Autodesk Inventor part; units mm, degrees
(part 2 of 3)
sketch "Sketch14" plane through (0, 0, 0) normal (0, 1, 0) x (1, 0, 0)
  line L0 (-0.8228, 6.9318) -> (-0.8228, 38.6692) construction
  line L1 (-0.8228, 38.6692) -> (1.7801, 38.6692) construction
  line L2 (1.7801, 38.6692) -> (1.7801, 6.9318) construction
  line L3 (1.7801, 6.9318) -> (-0.8228, 6.9318) construction
  line L4 (-3.7716, 9.8924) -> (-3.7716, 35.0917) construction
  line L5 (-3.7716, 35.0917) -> (-1.431, 35.0917) construction
  line L6 (-1.431, 35.0917) -> (-1.431, 9.8924) construction
  line L7 (-1.431, 9.8924) -> (-3.7716, 9.8924) construction
  spline S0 degree 2 poles (-1.6938, 10.6525) (-1.6938, 10.4354) (-1.7845, 10.1307) (-1.8494, 9.9961) knots 0 0 0 1 2 2 2
  line L8 (-1.8494, 9.9961) -> (-2.1832, 9.9961)
  line L9 (-2.1832, 9.9961) -> (-2.1832, 10.0156)
  spline S1 degree 2 poles (-2.1832, 10.0156) (-2.06, 10.1469) (-1.9239, 10.4791) (-1.9239, 10.6331) knots 0 0 0 1 2 2 2
  spline S2 degree 2 poles (-1.9239, 10.6331) (-1.9239, 10.8535) (-2.1071, 11.0788) (-2.2578, 11.0788) knots 0 0 0 1 2 2 2
  spline S3 degree 2 poles (-2.2578, 11.0788) (-2.3777, 11.0788) (-2.5268, 10.9605) (-2.5641, 10.8324) knots 0 0 0 1 2 2 2
  spline S4 degree 2 poles (-2.5641, 10.8324) (-2.59, 10.7401) (-2.6257, 10.5861) (-2.6549, 10.471) knots 0 0 0 1 2 2 2
  spline S5 degree 2 poles (-2.6549, 10.471) (-2.6824, 10.3673) (-2.7651, 10.2036) (-2.8315, 10.1404) knots 0 0 0 1 2 2 2
  spline S6 degree 2 poles (-2.8315, 10.1404) (-2.898, 10.0788) (-3.0763, 10.0107) (-3.193, 10.0107) knots 0 0 0 1 2 2 2
  spline S7 degree 2 poles (-3.193, 10.0107) (-3.4361, 10.0107) (-3.7651, 10.39) (-3.7651, 10.6833) knots 0 0 0 1 2 2 2
  spline S8 degree 2 poles (-3.7651, 10.6833) (-3.7651, 10.8519) (-3.6986, 11.1501) (-3.6354, 11.2781) knots 0 0 0 1 2 2 2
  line L10 (-3.6354, 11.2781) -> (-3.3177, 11.2781)
  line L11 (-3.3177, 11.2781) -> (-3.3177, 11.2587)
  spline S9 degree 2 poles (-3.3177, 11.2587) (-3.4053, 11.1631) (-3.5349, 10.8649) (-3.5349, 10.7012) knots 0 0 0 1 2 2 2
  spline S10 degree 2 poles (-3.5349, 10.7012) (-3.5349, 10.5164) (-3.3615, 10.2879) (-3.2205, 10.2879) knots 0 0 0 1 2 2 2
  spline S11 degree 2 poles (-3.2205, 10.2879) (-3.0941, 10.2879) (-2.9434, 10.4224) (-2.9093, 10.5488) knots 0 0 0 1 2 2 2
  spline S12 degree 2 poles (-2.9093, 10.5488) (-2.8866, 10.6331) (-2.8283, 10.8778) (-2.804, 10.9589) knots 0 0 0 1 2 2 2
  spline S13 degree 2 poles (-2.804, 10.9589) (-2.7408, 11.1647) (-2.4863, 11.3559) (-2.2999, 11.3559) knots 0 0 0 1 2 2 2
  spline S14 degree 2 poles (-2.2999, 11.3559) (-2.1816, 11.3559) (-1.9547, 11.2603) (-1.8753, 11.1744) knots 0 0 0 1 2 2 2
  spline S15 degree 2 poles (-1.8753, 11.1744) (-1.7878, 11.0788) (-1.6938, 10.8357) (-1.6938, 10.6525) knots 0 0 0 1 2 2 2
  line L12 (-1.7294, 12.3235) -> (-1.7294, 11.5488)
  line L13 (-1.7294, 11.5488) -> (-1.9336, 11.5488)
  line L14 (-1.9336, 11.5488) -> (-1.9336, 11.8033)
  line L15 (-1.9336, 11.8033) -> (-3.5252, 11.8033)
  line L16 (-3.5252, 11.8033) -> (-3.5252, 11.5488)
  line L17 (-3.5252, 11.5488) -> (-3.7294, 11.5488)
  line L18 (-3.7294, 11.5488) -> (-3.7294, 12.3235)
  line L19 (-3.7294, 12.3235) -> (-3.5252, 12.3235)
  line L20 (-3.5252, 12.3235) -> (-3.5252, 12.0691)
  line L21 (-3.5252, 12.0691) -> (-1.9336, 12.0691)
  line L22 (-1.9336, 12.0691) -> (-1.9336, 12.3235)
  line L23 (-1.9336, 12.3235) -> (-1.7294, 12.3235)
  line L24 (-3.7294, 14.894) -> (-1.7294, 14.3916)
  line L25 (-1.7294, 14.3916) -> (-1.7294, 14.0934)
  line L26 (-1.7294, 14.0934) -> (-3.3891, 13.6866)
  line L27 (-3.3891, 13.6866) -> (-1.7294, 13.2911)
  line L28 (-1.7294, 13.2911) -> (-1.7294, 12.9961)
  line L29 (-1.7294, 12.9961) -> (-3.7294, 12.4856)
  line L30 (-3.7294, 12.4856) -> (-3.7294, 12.7595)
  line L31 (-3.7294, 12.7595) -> (-2.0714, 13.1615)
  line L32 (-2.0714, 13.1615) -> (-3.7294, 13.5602)
  line L33 (-3.7294, 13.5602) -> (-3.7294, 13.8308)
  line L34 (-3.7294, 13.8308) -> (-2.0519, 14.2328)
  line L35 (-2.0519, 14.2328) -> (-3.7294, 14.6331)
  line L36 (-3.7294, 14.6331) -> (-3.7294, 14.894)
  line L37 (-1.7294, 14.9167) -> (-3.7294, 15.5909)
  line L38 (-3.7294, 15.5909) -> (-3.7294, 15.9183)
  line L39 (-3.7294, 15.9183) -> (-1.7294, 16.5926)
  line L40 (-1.7294, 16.5926) -> (-1.7294, 16.3122)
  line L41 (-1.7294, 16.3122) -> (-2.2886, 16.1307)
  line L42 (-2.2886, 16.1307) -> (-2.2886, 15.3673)
  line L43 (-2.2886, 15.3673) -> (-1.7294, 15.1858)
  line L44 (-1.7294, 15.1858) -> (-1.7294, 14.9167)
  line L45 (-2.5155, 16.0577) -> (-3.4571, 15.7482)
  line L46 (-3.4571, 15.7482) -> (-2.5155, 15.4402)
  line L47 (-2.5155, 15.4402) -> (-2.5155, 16.0577)
  line L48 (-1.7294, 17.249) -> (-3.4928, 17.249)
  line L49 (-3.4928, 17.249) -> (-3.4928, 16.578)
  line L50 (-3.4928, 16.578) -> (-3.7294, 16.578)
  line L51 (-3.7294, 16.578) -> (-3.7294, 18.1858)
  line L52 (-3.7294, 18.1858) -> (-3.4928, 18.1858)
  line L53 (-3.4928, 18.1858) -> (-3.4928, 17.5148)
  line L54 (-3.4928, 17.5148) -> (-1.7294, 17.5148)
  line L55 (-1.7294, 17.5148) -> (-1.7294, 17.249)
  line L56 (-1.7294, 19.9443) -> (-1.7294, 19.1696)
  line L57 (-1.7294, 19.1696) -> (-1.9336, 19.1696)
  line L58 (-1.9336, 19.1696) -> (-1.9336, 19.424)
  line L59 (-1.9336, 19.424) -> (-3.5252, 19.424)
  line L60 (-3.5252, 19.424) -> (-3.5252, 19.1696)
  line L61 (-3.5252, 19.1696) -> (-3.7294, 19.1696)
  line L62 (-3.7294, 19.1696) -> (-3.7294, 19.9443)
  line L63 (-3.7294, 19.9443) -> (-3.5252, 19.9443)
  line L64 (-3.5252, 19.9443) -> (-3.5252, 19.6898)
  line L65 (-3.5252, 19.6898) -> (-1.9336, 19.6898)
  line L66 (-1.9336, 19.6898) -> (-1.9336, 19.9443)
  line L67 (-1.9336, 19.9443) -> (-1.7294, 19.9443)
  line L68 (-1.7294, 21.7044) -> (-1.7294, 21.4062)
  line L69 (-1.7294, 21.4062) -> (-3.4539, 20.5213)
  line L70 (-3.4539, 20.5213) -> (-1.7294, 20.5213)
  line L71 (-1.7294, 20.5213) -> (-1.7294, 20.2733)
  line L72 (-1.7294, 20.2733) -> (-3.7294, 20.2733)
  line L73 (-3.7294, 20.2733) -> (-3.7294, 20.6509)
  line L74 (-3.7294, 20.6509) -> (-2.1459, 21.4564)
  line L75 (-2.1459, 21.4564) -> (-3.7294, 21.4564)
  line L76 (-3.7294, 21.4564) -> (-3.7294, 21.7044)
  line L77 (-3.7294, 21.7044) -> (-1.7294, 21.7044)
  spline S16 degree 2 poles (-1.6938, 22.8908) (-1.6938, 22.6963) (-1.825, 22.3673) (-1.9563, 22.2473) knots 0 0 0 1 2 2 2
  spline S17 degree 2 poles (-1.9563, 22.2473) (-2.086, 22.1274) (-2.475, 21.9961) (-2.7278, 21.9961) knots 0 0 0 1 2 2 2
  spline S18 degree 2 poles (-2.7278, 21.9961) (-2.979, 21.9961) (-3.3518, 22.1242) (-3.4895, 22.2457) knots 0 0 0 1 2 2 2
  spline S19 degree 2 poles (-3.4895, 22.2457) (-3.6241, 22.3657) (-3.7651, 22.6931) (-3.7651, 22.8956) knots 0 0 0 1 2 2 2
  spline S20 degree 2 poles (-3.7651, 22.8956) (-3.7651, 22.9961) (-3.7359, 23.1728) (-3.7132, 23.2473) knots 0 0 0 1 2 2 2
  spline S21 degree 2 poles (-3.7132, 23.2473) (-3.6921, 23.3122) (-3.6322, 23.4467) (-3.5965, 23.5132) knots 0 0 0 1 2 2 2
  line L78 (-3.5965, 23.5132) -> (-3.2756, 23.5132)
  line L79 (-3.2756, 23.5132) -> (-3.2756, 23.4921)
  spline S22 degree 2 poles (-3.2756, 23.4921) (-3.308, 23.4564) (-3.3988, 23.3462) (-3.4425, 23.2668) knots 0 0 0 1 2 2 2
  spline S23 degree 2 poles (-3.4425, 23.2668) (-3.4847, 23.1906) (-3.5382, 23.0107) (-3.5382, 22.894) knots 0 0 0 1 2 2 2
  spline S24 degree 2 poles (-3.5382, 22.894) (-3.5382, 22.766) (-3.4328, 22.5375) (-3.3323, 22.4516) knots 0 0 0 1 2 2 2
  spline S25 degree 2 poles (-3.3323, 22.4516) (-3.2302, 22.3673) (-2.9207, 22.2733) (-2.7278, 22.2733) knots 0 0 0 1 2 2 2
  spline S26 degree 2 poles (-2.7278, 22.2733) (-2.522, 22.2733) (-2.2254, 22.3721) (-2.1233, 22.458) knots 0 0 0 1 2 2 2
  spline S27 degree 2 poles (-2.1233, 22.458) (-2.0244, 22.5423) (-1.9239, 22.7676) (-1.9239, 22.894) knots 0 0 0 1 2 2 2
  spline S28 degree 2 poles (-1.9239, 22.894) (-1.9239, 23.0091) (-1.9806, 23.2052) (-2.0228, 23.2814) knots 0 0 0 1 2 2 2
  spline S29 degree 2 poles (-2.0228, 23.2814) (-2.0649, 23.3543) (-2.1524, 23.4629) (-2.1832, 23.4937) knots 0 0 0 1 2 2 2
  line L80 (-2.1832, 23.4937) -> (-2.1832, 23.5132)
  line L81 (-2.1832, 23.5132) -> (-1.8656, 23.5132)
  spline S30 degree 2 poles (-1.8656, 23.5132) (-1.8348, 23.4467) (-1.778, 23.33) (-1.7521, 23.2473) knots 0 0 0 1 2 2 2
  spline S31 degree 2 poles (-1.7521, 23.2473) (-1.7229, 23.1598) (-1.6938, 23.0107) (-1.6938, 22.8908) knots 0 0 0 1 2 2 2
  spline S32 degree 2 poles (-1.24, 26.2814) (-1.2221, 26.2085) (-1.2027, 26.0496) (-1.2027, 25.9702) knots 0 0 0 1 2 2 2
  spline S33 degree 2 poles (-1.2027, 25.9702) (-1.2027, 25.7449) (-1.4539, 25.4645) (-1.6873, 25.4516) knots 0 0 0 1 2 2 2
  spline S34 degree 2 poles (-1.6873, 25.4516) (-1.6873, 25.4337) (-1.6873, 25.4029) (-1.6873, 25.39) knots 0 0 0 1 2 2 2
  spline S35 degree 2 poles (-1.6873, 25.39) (-1.6873, 25.1874) (-1.825, 24.8616) (-1.9596, 24.7449) knots 0 0 0 1 2 2 2
  spline S36 degree 2 poles (-1.9596, 24.7449) (-2.0925, 24.6298) (-2.4814, 24.5067) (-2.7278, 24.5067) knots 0 0 0 1 2 2 2
  spline S37 degree 2 poles (-2.7278, 24.5067) (-2.9806, 24.5067) (-3.3631, 24.6315) (-3.4993, 24.7465) knots 0 0 0 1 2 2 2
  spline S38 degree 2 poles (-3.4993, 24.7465) (-3.6338, 24.8632) (-3.7716, 25.189) (-3.7716, 25.39) knots 0 0 0 1 2 2 2
  spline S39 degree 2 poles (-3.7716, 25.39) (-3.7716, 25.5942) (-3.6289, 25.9216) (-3.4993, 26.035) knots 0 0 0 1 2 2 2
  spline S40 degree 2 poles (-3.4993, 26.035) (-3.368, 26.1485) (-2.9774, 26.2749) (-2.7278, 26.2749) knots 0 0 0 1 2 2 2
  spline S41 degree 2 poles (-2.7278, 26.2749) (-2.3388, 26.2749) (-1.8331, 25.9718) (-1.744, 25.7076) knots 0 0 0 1 2 2 2
  spline S42 degree 2 poles (-1.744, 25.7076) (-1.6694, 25.7141) (-1.5495, 25.753) (-1.5155, 25.7838) knots 0 0 0 1 2 2 2
  spline S43 degree 2 poles (-1.5155, 25.7838) (-1.4733, 25.8211) (-1.4344, 25.9232) (-1.4344, 26.014) knots 0 0 0 1 2 2 2
  spline S44 degree 2 poles (-1.4344, 26.014) (-1.4344, 26.0674) (-1.4685, 26.2133) (-1.4814, 26.2457) knots 0 0 0 1 2 2 2
  line L82 (-1.4814, 26.2457) -> (-1.4814, 26.2814)
  line L83 (-1.4814, 26.2814) -> (-1.24, 26.2814)
  spline S45 degree 2 poles (-2.7278, 25.9978) (-2.9271, 25.9978) (-3.2335, 25.9119) (-3.334, 25.8341) knots 0 0 0 1 2 2 2
  spline S46 degree 2 poles (-3.334, 25.8341) (-3.4377, 25.7546) (-3.5414, 25.531) (-3.5414, 25.3916) knots 0 0 0 1 2 2 2
  spline S47 degree 2 poles (-3.5414, 25.3916) (-3.5414, 25.2473) (-3.4409, 25.0302) (-3.334, 24.9475) knots 0 0 0 1 2 2 2
  spline S48 degree 2 poles (-3.334, 24.9475) (-3.2318, 24.8681) (-2.9223, 24.7838) (-2.7278, 24.7838) knots 0 0 0 1 2 2 2
  spline S49 degree 2 poles (-2.7278, 24.7838) (-2.334, 24.7838) (-1.9142, 25.1144) (-1.9142, 25.3916) knots 0 0 0 1 2 2 2
  spline S50 degree 2 poles (-1.9142, 25.3916) (-1.9142, 25.6687) (-2.334, 25.9978) (-2.7278, 25.9978) knots 0 0 0 1 2 2 2
  spline S51 degree 2 poles (-3.5398, 27.0496) (-3.5398, 26.9767) (-3.5041, 26.8324) (-3.4766, 26.7627) knots 0 0 0 1 2 2 2
  spline S52 degree 2 poles (-3.4766, 26.7627) (-3.449, 26.6979) (-3.3907, 26.6023) (-3.3647, 26.565) knots 0 0 0 1 2 2 2
  line L84 (-3.3647, 26.565) -> (-3.3647, 26.5488)
  line L85 (-3.3647, 26.5488) -> (-3.6484, 26.5488)
  spline S53 degree 2 poles (-3.6484, 26.5488) (-3.6954, 26.6363) (-3.7716, 26.9362) (-3.7716, 27.0707) knots 0 0 0 1 2 2 2
  spline S54 degree 2 poles (-3.7716, 27.0707) (-3.7716, 27.2068) (-3.7165, 27.4094) (-3.6581, 27.4921) knots 0 0 0 1 2 2 2
  spline S55 degree 2 poles (-3.6581, 27.4921) (-3.5949, 27.5796) (-3.4118, 27.6704) (-3.2886, 27.6704) knots 0 0 0 1 2 2 2
  spline S56 degree 2 poles (-3.2886, 27.6704) (-3.1233, 27.6704) (-2.8737, 27.4532) (-2.8412, 27.3008) knots 0 0 0 1 2 2 2
  line L86 (-2.8412, 27.3008) -> (-2.8218, 27.3008)
  spline S57 degree 2 poles (-2.8218, 27.3008) (-2.8088, 27.364) (-2.7505, 27.5083) (-2.6921, 27.5699) knots 0 0 0 1 2 2 2
  spline S58 degree 2 poles (-2.6921, 27.5699) (-2.6354, 27.6315) (-2.4539, 27.7093) (-2.3226, 27.7093) knots 0 0 0 1 2 2 2
  spline S59 degree 2 poles (-2.3226, 27.7093) (-2.1881, 27.7093) (-1.9596, 27.6169) (-1.872, 27.5326) knots 0 0 0 1 2 2 2
  spline S60 degree 2 poles (-1.872, 27.5326) (-1.7813, 27.4451) (-1.6873, 27.1971) (-1.6873, 27.0399) knots 0 0 0 1 2 2 2
  spline S61 degree 2 poles (-1.6873, 27.0399) (-1.6873, 26.8892) (-1.7602, 26.5942) (-1.8105, 26.4937) knots 0 0 0 1 2 2 2
  line L87 (-1.8105, 26.4937) -> (-2.0941, 26.4937)
  line L88 (-2.0941, 26.4937) -> (-2.0941, 26.5132)
  spline S62 degree 2 poles (-2.0941, 26.5132) (-2.0325, 26.5974) (-1.919, 26.8827) (-1.919, 27.0237) knots 0 0 0 1 2 2 2
  spline S63 degree 2 poles (-1.919, 27.0237) (-1.919, 27.1063) (-1.9709, 27.2717) (-2.0309, 27.3268) knots 0 0 0 1 2 2 2
  spline S64 degree 2 poles (-2.0309, 27.3268) (-2.0908, 27.3803) (-2.2335, 27.437) (-2.3421, 27.437) knots 0 0 0 1 2 2 2
  spline S65 degree 2 poles (-2.3421, 27.437) (-2.4506, 27.437) (-2.5917, 27.3738) (-2.6322, 27.317) knots 0 0 0 1 2 2 2
  spline S66 degree 2 poles (-2.6322, 27.317) (-2.6727, 27.2603) (-2.7035, 27.1063) (-2.7035, 27.0156) knots 0 0 0 1 2 2 2
  line L89 (-2.7035, 27.0156) -> (-2.7035, 26.9021)
  line L90 (-2.7035, 26.9021) -> (-2.9255, 26.9021)
  line L91 (-2.9255, 26.9021) -> (-2.9255, 26.9913)
  spline S67 degree 2 poles (-2.9255, 26.9913) (-2.9255, 27.1712) (-3.0973, 27.3981) (-3.261, 27.3981) knots 0 0 0 1 2 2 2
  spline S68 degree 2 poles (-3.261, 27.3981) (-3.3372, 27.3981) (-3.4458, 27.3397) (-3.4782, 27.2927) knots 0 0 0 1 2 2 2
  spline S69 degree 2 poles (-3.4782, 27.2927) (-3.5122, 27.2425) (-3.5398, 27.1193) (-3.5398, 27.0496) knots 0 0 0 1 2 2 2
  line L92 (-1.7294, 30.1031) -> (-1.7294, 28.8697)
  line L93 (-1.7294, 28.8697) -> (-2.013, 28.8697)
  spline S70 degree 2 poles (-2.013, 28.8697) (-2.1378, 29.0026) (-2.3696, 29.2392) (-2.4944, 29.3527) knots 0 0 0 1 2 2 2
  spline S71 degree 2 poles (-2.4944, 29.3527) (-2.7456, 29.5812) (-3.0471, 29.7482) (-3.2075, 29.7482) knots 0 0 0 1 2 2 2
  spline S72 degree 2 poles (-3.2075, 29.7482) (-3.2918, 29.7482) (-3.4182, 29.6963) (-3.4588, 29.6493) knots 0 0 0 1 2 2 2
  spline S73 degree 2 poles (-3.4588, 29.6493) (-3.4993, 29.6023) (-3.5398, 29.4791) (-3.5398, 29.4046) knots 0 0 0 1 2 2 2
  spline S74 degree 2 poles (-3.5398, 29.4046) (-3.5398, 29.3332) (-3.5041, 29.1874) (-3.4766, 29.1209) knots 0 0 0 1 2 2 2
  spline S75 degree 2 poles (-3.4766, 29.1209) (-3.4539, 29.0642) (-3.3891, 28.9589) (-3.3664, 28.9264) knots 0 0 0 1 2 2 2
  line L94 (-3.3664, 28.9264) -> (-3.3664, 28.9119)
  line L95 (-3.3664, 28.9119) -> (-3.6516, 28.9119)
  spline S76 degree 2 poles (-3.6516, 28.9119) (-3.6921, 28.9945) (-3.7716, 29.2911) (-3.7716, 29.424) knots 0 0 0 1 2 2 2
  spline S77 degree 2 poles (-3.7716, 29.424) (-3.7716, 29.7044) (-3.475, 30.0204) (-3.2221, 30.0204) knots 0 0 0 1 2 2 2
  spline S78 degree 2 poles (-3.2221, 30.0204) (-3.1038, 30.0204) (-2.9061, 29.9653) (-2.8218, 29.9167) knots 0 0 0 1 2 2 2
  spline S79 degree 2 poles (-2.8218, 29.9167) (-2.7343, 29.8681) (-2.5625, 29.7271) (-2.4798, 29.6493) knots 0 0 0 1 2 2 2
  spline S80 degree 2 poles (-2.4798, 29.6493) (-2.3421, 29.5229) (-2.0471, 29.2133) (-1.9612, 29.1209) knots 0 0 0 1 2 2 2
  line L96 (-1.9612, 29.1209) -> (-1.9612, 30.1031)
  line L97 (-1.9612, 30.1031) -> (-1.7294, 30.1031)
  spline S81 degree 2 poles (-2.7294, 31.6153) (-2.1913, 31.6153) (-1.6873, 31.3025) (-1.6873, 30.9767) knots 0 0 0 1 2 2 2
  spline S82 degree 2 poles (-1.6873, 30.9767) (-1.6873, 30.6461) (-2.2011, 30.3365) (-2.7278, 30.3365) knots 0 0 0 1 2 2 2
  spline S83 degree 2 poles (-2.7278, 30.3365) (-3.2691, 30.3365) (-3.7699, 30.6493) (-3.7699, 30.9767) knots 0 0 0 1 2 2 2
  spline S84 degree 2 poles (-3.7699, 30.9767) (-3.7699, 31.3057) (-3.2513, 31.6153) (-2.7294, 31.6153) knots 0 0 0 1 2 2 2
  spline S85 degree 2 poles (-2.12, 31.2717) (-2.2189, 31.3106) (-2.5236, 31.343) (-2.7294, 31.343) knots 0 0 0 1 2 2 2
  spline S86 degree 2 poles (-2.7294, 31.343) (-2.9353, 31.343) (-3.2383, 31.3106) (-3.3404, 31.27) knots 0 0 0 1 2 2 2
  spline S87 degree 2 poles (-3.3404, 31.27) (-3.4425, 31.2295) (-3.5479, 31.0885) (-3.5479, 30.9767) knots 0 0 0 1 2 2 2
  spline S88 degree 2 poles (-3.5479, 30.9767) (-3.5479, 30.8649) (-3.4425, 30.7206) (-3.3372, 30.6785) knots 0 0 0 1 2 2 2
  spline S89 degree 2 poles (-3.3372, 30.6785) (-3.2351, 30.6379) (-2.9239, 30.6088) (-2.7278, 30.6088) knots 0 0 0 1 2 2 2
  spline S90 degree 2 poles (-2.7278, 30.6088) (-2.5171, 30.6088) (-2.2351, 30.6347) (-2.1249, 30.6768) knots 0 0 0 1 2 2 2
  spline S91 degree 2 poles (-2.1249, 30.6768) (-2.0212, 30.7157) (-1.9093, 30.86) (-1.9093, 30.9767) knots 0 0 0 1 2 2 2
  spline S92 degree 2 poles (-1.9093, 30.9767) (-1.9093, 31.0869) (-2.0147, 31.2311) (-2.12, 31.2717) knots 0 0 0 1 2 2 2
  line L98 (-1.7294, 33.1047) -> (-1.7294, 31.8713)
  line L99 (-1.7294, 31.8713) -> (-2.013, 31.8713)
  spline S93 degree 2 poles (-2.013, 31.8713) (-2.1378, 32.0042) (-2.3696, 32.2409) (-2.4944, 32.3543) knots 0 0 0 1 2 2 2
  spline S94 degree 2 poles (-2.4944, 32.3543) (-2.7456, 32.5828) (-3.0471, 32.7498) (-3.2075, 32.7498) knots 0 0 0 1 2 2 2
  spline S95 degree 2 poles (-3.2075, 32.7498) (-3.2918, 32.7498) (-3.4182, 32.6979) (-3.4588, 32.6509) knots 0 0 0 1 2 2 2
  spline S96 degree 2 poles (-3.4588, 32.6509) (-3.4993, 32.6039) (-3.5398, 32.4807) (-3.5398, 32.4062) knots 0 0 0 1 2 2 2
  spline S97 degree 2 poles (-3.5398, 32.4062) (-3.5398, 32.3349) (-3.5041, 32.189) (-3.4766, 32.1226) knots 0 0 0 1 2 2 2
  spline S98 degree 2 poles (-3.4766, 32.1226) (-3.4539, 32.0658) (-3.3891, 31.9605) (-3.3664, 31.9281) knots 0 0 0 1 2 2 2
  line L100 (-3.3664, 31.9281) -> (-3.3664, 31.9135)
  line L101 (-3.3664, 31.9135) -> (-3.6516, 31.9135)
  spline S99 degree 2 poles (-3.6516, 31.9135) (-3.6921, 31.9961) (-3.7716, 32.2927) (-3.7716, 32.4256) knots 0 0 0 1 2 2 2
  spline S100 degree 2 poles (-3.7716, 32.4256) (-3.7716, 32.706) (-3.475, 33.0221) (-3.2221, 33.0221) knots 0 0 0 1 2 2 2
  spline S101 degree 2 poles (-3.2221, 33.0221) (-3.1038, 33.0221) (-2.9061, 32.967) (-2.8218, 32.9183) knots 0 0 0 1 2 2 2
  spline S102 degree 2 poles (-2.8218, 32.9183) (-2.7343, 32.8697) (-2.5625, 32.7287) (-2.4798, 32.6509) knots 0 0 0 1 2 2 2
  spline S103 degree 2 poles (-2.4798, 32.6509) (-2.3421, 32.5245) (-2.0471, 32.2149) (-1.9612, 32.1226) knots 0 0 0 1 2 2 2
  line L102 (-1.9612, 32.1226) -> (-1.9612, 33.1047)
  line L103 (-1.9612, 33.1047) -> (-1.7294, 33.1047)
  line L104 (-1.7294, 34.6055) -> (-1.7294, 33.3721)
  line L105 (-1.7294, 33.3721) -> (-2.013, 33.3721)
  spline S104 degree 2 poles (-2.013, 33.3721) (-2.1378, 33.505) (-2.3696, 33.7417) (-2.4944, 33.8551) knots 0 0 0 1 2 2 2
  spline S105 degree 2 poles (-2.4944, 33.8551) (-2.7456, 34.0837) (-3.0471, 34.2506) (-3.2075, 34.2506) knots 0 0 0 1 2 2 2
  spline S106 degree 2 poles (-3.2075, 34.2506) (-3.2918, 34.2506) (-3.4182, 34.1987) (-3.4588, 34.1517) knots 0 0 0 1 2 2 2
  spline S107 degree 2 poles (-3.4588, 34.1517) (-3.4993, 34.1047) (-3.5398, 33.9815) (-3.5398, 33.907) knots 0 0 0 1 2 2 2
  spline S108 degree 2 poles (-3.5398, 33.907) (-3.5398, 33.8357) (-3.5041, 33.6898) (-3.4766, 33.6234) knots 0 0 0 1 2 2 2
  spline S109 degree 2 poles (-3.4766, 33.6234) (-3.4539, 33.5666) (-3.3891, 33.4613) (-3.3664, 33.4289) knots 0 0 0 1 2 2 2
  line L106 (-3.3664, 33.4289) -> (-3.3664, 33.4143)
  line L107 (-3.3664, 33.4143) -> (-3.6516, 33.4143)
  spline S110 degree 2 poles (-3.6516, 33.4143) (-3.6921, 33.4969) (-3.7716, 33.7935) (-3.7716, 33.9264) knots 0 0 0 1 2 2 2
  spline S111 degree 2 poles (-3.7716, 33.9264) (-3.7716, 34.2068) (-3.475, 34.5229) (-3.2221, 34.5229) knots 0 0 0 1 2 2 2
  spline S112 degree 2 poles (-3.2221, 34.5229) (-3.1038, 34.5229) (-2.9061, 34.4678) (-2.8218, 34.4191) knots 0 0 0 1 2 2 2
  spline S113 degree 2 poles (-2.8218, 34.4191) (-2.7343, 34.3705) (-2.5625, 34.2295) (-2.4798, 34.1517) knots 0 0 0 1 2 2 2
  spline S114 degree 2 poles (-2.4798, 34.1517) (-2.3421, 34.0253) (-2.0471, 33.7157) (-1.9612, 33.6234) knots 0 0 0 1 2 2 2
  line L108 (-1.9612, 33.6234) -> (-1.9612, 34.6055)
  line L109 (-1.9612, 34.6055) -> (-1.7294, 34.6055)
  spline S115 degree 2 poles (-0.1842, 8.3986) (-0.0546, 8.3986) (0.1788, 8.3062) (0.2599, 8.2235) knots 0 0 0 1 2 2 2
  spline S116 degree 2 poles (0.2599, 8.2235) (0.362, 8.1198) (0.4673, 7.8394) (0.4673, 7.6255) knots 0 0 0 1 2 2 2
  line L110 (0.4673, 7.6255) -> (0.4673, 7.4002)
  line L111 (0.4673, 7.4002) -> (1.2129, 7.4002)
  line L112 (1.2129, 7.4002) -> (1.2129, 7.1344)
  line L113 (1.2129, 7.1344) -> (-0.7871, 7.1344)
  line L114 (-0.7871, 7.1344) -> (-0.7871, 7.6368)
  spline S117 degree 2 poles (-0.7871, 7.6368) (-0.7871, 7.8151) (-0.7288, 8.0647) (-0.6623, 8.1603) knots 0 0 0 1 2 2 2
  spline S118 degree 2 poles (-0.6623, 8.1603) (-0.5862, 8.2721) (-0.3512, 8.3986) (-0.1842, 8.3986) knots 0 0 0 1 2 2 2
  spline S119 degree 2 poles (-0.1761, 8.1214) (-0.2799, 8.1214) (-0.4322, 8.0501) (-0.4808, 7.9772) knots 0 0 0 1 2 2 2
  spline S120 degree 2 poles (-0.4808, 7.9772) (-0.523, 7.914) (-0.557, 7.7454) (-0.557, 7.6206) knots 0 0 0 1 2 2 2
  line L115 (-0.557, 7.6206) -> (-0.557, 7.4002)
  line L116 (-0.557, 7.4002) -> (0.2404, 7.4002)
  line L117 (0.2404, 7.4002) -> (0.2404, 7.5817)
  spline S121 degree 2 poles (0.2404, 7.5817) (0.2404, 7.7438) (0.1885, 7.9431) (0.1205, 8.008) knots 0 0 0 1 2 2 2
  spline S122 degree 2 poles (0.1205, 8.008) (0.0605, 8.0679) (-0.0805, 8.1214) (-0.1761, 8.1214) knots 0 0 0 1 2 2 2
  line L118 (-0.0173, 9.4277) -> (-0.0173, 9.4148)
  spline S123 degree 2 poles (-0.0173, 9.4148) (-0.0254, 9.3856) (-0.0286, 9.3224) (-0.0286, 9.2786) knots 0 0 0 1 2 2 2
  spline S124 degree 2 poles (-0.0286, 9.2786) (-0.0286, 9.1765) (0.0605, 8.9755) (0.148, 8.8848) knots 0 0 0 1 2 2 2
  line L119 (0.148, 8.8848) -> (1.2129, 8.8848)
  line L120 (1.2129, 8.8848) -> (1.2129, 8.6319)
  line L121 (1.2129, 8.6319) -> (-0.288, 8.6319)
  line L122 (-0.288, 8.6319) -> (-0.288, 8.8848)
  line L123 (-0.288, 8.8848) -> (-0.0643, 8.8848)
  spline S125 degree 2 poles (-0.0643, 8.8848) (-0.1875, 9.0225) (-0.288, 9.2284) (-0.288, 9.3256) knots 0 0 0 1 2 2 2
  spline S126 degree 2 poles (-0.288, 9.3256) (-0.288, 9.3645) (-0.2847, 9.4034) (-0.2799, 9.4277) knots 0 0 0 1 2 2 2
  line L124 (-0.2799, 9.4277) -> (-0.0173, 9.4277)
  spline S127 degree 2 poles (0.4624, 10.8572) (0.8417, 10.8572) (1.255, 10.4926) (1.255, 10.1879) knots 0 0 0 1 2 2 2
  spline S128 degree 2 poles (1.255, 10.1879) (1.255, 9.8751) (0.8287, 9.5169) (0.4624, 9.5169) knots 0 0 0 1 2 2 2
  spline S129 degree 2 poles (0.4624, 9.5169) (0.0864, 9.5169) (-0.3301, 9.8864) (-0.3301, 10.1879) knots 0 0 0 1 2 2 2
  spline S130 degree 2 poles (-0.3301, 10.1879) (-0.3301, 10.4926) (0.0848, 10.8572) (0.4624, 10.8572) knots 0 0 0 1 2 2 2
  spline S131 degree 2 poles (0.4624, 10.5963) (0.1707, 10.5963) (-0.1129, 10.384) (-0.1129, 10.1879) knots 0 0 0 1 2 2 2
  spline S132 degree 2 poles (-0.1129, 10.1879) (-0.1129, 9.9917) (0.1707, 9.7778) (0.4624, 9.7778) knots 0 0 0 1 2 2 2
  spline S133 degree 2 poles (0.4624, 9.7778) (0.7461, 9.7778) (1.0378, 9.9917) (1.0378, 10.1879) knots 0 0 0 1 2 2 2
  spline S134 degree 2 poles (1.0378, 10.1879) (1.0378, 10.3823) (0.7509, 10.5963) (0.4624, 10.5963) knots 0 0 0 1 2 2 2
  spline S135 degree 2 poles (1.255, 11.525) (1.5111, 11.525) (1.7801, 11.2494) (1.7801, 11.008) knots 0 0 0 1 2 2 2
  spline S136 degree 2 poles (1.7801, 11.008) (1.7801, 10.9658) (1.772, 10.8621) (1.7639, 10.8118) knots 0 0 0 1 2 2 2
  line L125 (1.7639, 10.8118) -> (1.537, 10.8118)
  line L126 (1.537, 10.8118) -> (1.537, 10.8264)
  spline S137 degree 2 poles (1.537, 10.8264) (1.5435, 10.8556) (1.5565, 10.9269) (1.5565, 10.9593) knots 0 0 0 1 2 2 2
  spline S138 degree 2 poles (1.5565, 10.9593) (1.5565, 11.0598) (1.5062, 11.1911) (1.4527, 11.2219) knots 0 0 0 1 2 2 2
  spline S139 degree 2 poles (1.4527, 11.2219) (1.4041, 11.2527) (1.2566, 11.2721) (1.1513, 11.2721) knots 0 0 0 1 2 2 2
  line L127 (1.1513, 11.2721) -> (-0.0789, 11.2721)
  line L128 (-0.0789, 11.2721) -> (-0.0789, 11.0015)
  line L129 (-0.0789, 11.0015) -> (-0.288, 11.0015)
  line L130 (-0.288, 11.0015) -> (-0.288, 11.525)
  line L131 (-0.288, 11.525) -> (1.255, 11.525)
  line L132 (-0.5376, 11.5266) -> (-0.5376, 11.2397)
  line L133 (-0.5376, 11.2397) -> (-0.8001, 11.2397)
  line L134 (-0.8001, 11.2397) -> (-0.8001, 11.5266)
  line L135 (-0.8001, 11.5266) -> (-0.5376, 11.5266)
  spline S140 degree 2 poles (1.2469, 12.5428) (1.2469, 12.183) (0.8433, 11.7875) (0.4706, 11.7875) knots 0 0 0 1 2 2 2
  spline S141 degree 2 poles (0.4706, 11.7875) (0.1043, 11.7875) (-0.3301, 12.1717) (-0.3301, 12.4812) knots 0 0 0 1 2 2 2
  spline S142 degree 2 poles (-0.3301, 12.4812) (-0.3301, 12.6206) (-0.2491, 12.8362) (-0.1632, 12.9156) knots 0 0 0 1 2 2 2
  spline S143 degree 2 poles (-0.1632, 12.9156) (-0.0773, 12.9966) (0.1707, 13.0825) (0.3506, 13.0825) knots 0 0 0 1 2 2 2
  line L136 (0.3506, 13.0825) -> (0.4884, 13.0825)
  line L137 (0.4884, 13.0825) -> (0.4884, 12.0436)
  spline S144 degree 2 poles (0.4884, 12.0436) (0.7493, 12.0436) (1.0265, 12.3062) (1.0265, 12.5396) knots 0 0 0 1 2 2 2
  spline S145 degree 2 poles (1.0265, 12.5396) (1.0265, 12.6222) (0.9892, 12.7827) (0.96, 12.8475) knots 0 0 0 1 2 2 2
  spline S146 degree 2 poles (0.96, 12.8475) (0.9276, 12.9156) (0.8709, 13.0096) (0.8449, 13.0404) knots 0 0 0 1 2 2 2
  line L138 (0.8449, 13.0404) -> (0.8449, 13.055)
  line L139 (0.8449, 13.055) -> (1.1205, 13.055)
  spline S147 degree 2 poles (1.1205, 13.055) (1.1383, 13.0112) (1.1902, 12.8783) (1.2047, 12.8264) knots 0 0 0 1 2 2 2
  spline S148 degree 2 poles (1.2047, 12.8264) (1.2258, 12.7535) (1.2469, 12.6336) (1.2469, 12.5428) knots 0 0 0 1 2 2 2
  spline S149 degree 2 poles (0.2955, 12.8362) (0.1934, 12.8329) (0.0443, 12.7908) (-0.0059, 12.7503) knots 0 0 0 1 2 2 2
  spline S150 degree 2 poles (-0.0059, 12.7503) (-0.0627, 12.7065) (-0.1226, 12.5687) (-0.1226, 12.4666) knots 0 0 0 1 2 2 2
  spline S151 degree 2 poles (-0.1226, 12.4666) (-0.1226, 12.3661) (-0.0627, 12.2251) (-0.0043, 12.1668) knots 0 0 0 1 2 2 2
  spline S152 degree 2 poles (-0.0043, 12.1668) (0.0556, 12.1101) (0.1999, 12.0517) (0.2955, 12.0436) knots 0 0 0 1 2 2 2
  line L140 (0.2955, 12.0436) -> (0.2955, 12.8362)
  spline S153 degree 2 poles (1.2469, 13.935) (1.2469, 13.7794) (1.1513, 13.5217) (1.054, 13.4294) knots 0 0 0 1 2 2 2
  spline S154 degree 2 poles (1.054, 13.4294) (0.9584, 13.337) (0.6634, 13.2349) (0.4657, 13.2349) knots 0 0 0 1 2 2 2
  spline S155 degree 2 poles (0.4657, 13.2349) (0.268, 13.2349) (-0.0205, 13.3402) (-0.1178, 13.4294) knots 0 0 0 1 2 2 2
  spline S156 degree 2 poles (-0.1178, 13.4294) (-0.2166, 13.5185) (-0.322, 13.7827) (-0.322, 13.935) knots 0 0 0 1 2 2 2
  spline S157 degree 2 poles (-0.322, 13.935) (-0.322, 14.0582) (-0.2523, 14.2883) (-0.2069, 14.3775) knots 0 0 0 1 2 2 2
  line L141 (-0.2069, 14.3775) -> (0.0767, 14.3775)
  line L142 (0.0767, 14.3775) -> (0.0767, 14.3629)
  spline S158 degree 2 poles (0.0767, 14.3629) (0.054, 14.3353) (-0.0043, 14.2511) (-0.0351, 14.1911) knots 0 0 0 1 2 2 2
  spline S159 degree 2 poles (-0.0351, 14.1911) (-0.0611, 14.1376) (-0.1016, 13.995) (-0.1016, 13.9302) knots 0 0 0 1 2 2 2
  spline S160 degree 2 poles (-0.1016, 13.9302) (-0.1016, 13.7341) (0.195, 13.4958) (0.4657, 13.4958) knots 0 0 0 1 2 2 2
  spline S161 degree 2 poles (0.4657, 13.4958) (0.7299, 13.4958) (1.0265, 13.7259) (1.0265, 13.9302) knots 0 0 0 1 2 2 2
  spline S162 degree 2 poles (1.0265, 13.9302) (1.0265, 14.0533) (0.9244, 14.277) (0.8449, 14.3629) knots 0 0 0 1 2 2 2
  line L143 (0.8449, 14.3629) -> (0.8449, 14.3775)
  line L144 (0.8449, 14.3775) -> (1.1286, 14.3775)
  spline S163 degree 2 poles (1.1286, 14.3775) (1.1464, 14.3402) (1.1966, 14.2268) (1.208, 14.1814) knots 0 0 0 1 2 2 2
  spline S164 degree 2 poles (1.208, 14.1814) (1.2274, 14.1165) (1.2469, 14.0144) (1.2469, 13.935) knots 0 0 0 1 2 2 2
  spline S165 degree 2 poles (1.242, 15.0614) (1.242, 14.8556) (1.007, 14.6238) (0.7526, 14.6238) knots 0 0 0 1 2 2 2
  line L145 (0.7526, 14.6238) -> (-0.0789, 14.6238)
  line L146 (-0.0789, 14.6238) -> (-0.0789, 14.4537)
  line L147 (-0.0789, 14.4537) -> (-0.288, 14.4537)
  line L148 (-0.288, 14.4537) -> (-0.288, 14.6238)
  line L149 (-0.288, 14.6238) -> (-0.7191, 14.6238)
  line L150 (-0.7191, 14.6238) -> (-0.7191, 14.8767)
  line L151 (-0.7191, 14.8767) -> (-0.288, 14.8767)
  line L152 (-0.288, 14.8767) -> (-0.288, 15.3418)
  line L153 (-0.288, 15.3418) -> (-0.0789, 15.3418)
  line L154 (-0.0789, 15.3418) -> (-0.0789, 14.8767)
  line L155 (-0.0789, 14.8767) -> (0.6359, 14.8767)
  spline S166 degree 2 poles (0.6359, 14.8767) (0.7493, 14.8767) (0.8741, 14.8848) (0.9276, 14.9123) knots 0 0 0 1 2 2 2
  spline S167 degree 2 poles (0.9276, 14.9123) (0.9746, 14.935) (1.0216, 15.0371) (1.0216, 15.1246) knots 0 0 0 1 2 2 2
  spline S168 degree 2 poles (1.0216, 15.1246) (1.0216, 15.1862) (0.9843, 15.3013) (0.973, 15.3272) knots 0 0 0 1 2 2 2
  line L156 (0.973, 15.3272) -> (0.973, 15.3418)
  line L157 (0.973, 15.3418) -> (1.1999, 15.3418)
  spline S169 degree 2 poles (1.1999, 15.3418) (1.2193, 15.2705) (1.242, 15.1246) (1.242, 15.0614) knots 0 0 0 1 2 2 2
  spline S170 degree 2 poles (1.2485, 16.9642) (1.2485, 16.747) (1.1577, 16.4423) (1.0929, 16.3078) knots 0 0 0 1 2 2 2
  line L158 (1.0929, 16.3078) -> (0.759, 16.3078)
  line L159 (0.759, 16.3078) -> (0.759, 16.3272)
  spline S171 degree 2 poles (0.759, 16.3272) (0.8822, 16.4585) (1.0184, 16.7908) (1.0184, 16.9447) knots 0 0 0 1 2 2 2
  spline S172 degree 2 poles (1.0184, 16.9447) (1.0184, 17.1652) (0.8352, 17.3905) (0.6845, 17.3905) knots 0 0 0 1 2 2 2
  spline S173 degree 2 poles (0.6845, 17.3905) (0.5646, 17.3905) (0.4154, 17.2721) (0.3782, 17.1441) knots 0 0 0 1 2 2 2
  spline S174 degree 2 poles (0.3782, 17.1441) (0.3522, 17.0517) (0.3166, 16.8977) (0.2874, 16.7827) knots 0 0 0 1 2 2 2
  spline S175 degree 2 poles (0.2874, 16.7827) (0.2599, 16.6789) (0.1772, 16.5152) (0.1107, 16.452) knots 0 0 0 1 2 2 2
  spline S176 degree 2 poles (0.1107, 16.452) (0.0443, 16.3905) (-0.134, 16.3224) (-0.2507, 16.3224) knots 0 0 0 1 2 2 2
  spline S177 degree 2 poles (-0.2507, 16.3224) (-0.4938, 16.3224) (-0.8228, 16.7016) (-0.8228, 16.995) knots 0 0 0 1 2 2 2
  spline S178 degree 2 poles (-0.8228, 16.995) (-0.8228, 17.1635) (-0.7564, 17.4618) (-0.6931, 17.5898) knots 0 0 0 1 2 2 2
  line L160 (-0.6931, 17.5898) -> (-0.3755, 17.5898)
  line L161 (-0.3755, 17.5898) -> (-0.3755, 17.5704)
  spline S179 degree 2 poles (-0.3755, 17.5704) (-0.463, 17.4747) (-0.5927, 17.1765) (-0.5927, 17.0128) knots 0 0 0 1 2 2 2
  spline S180 degree 2 poles (-0.5927, 17.0128) (-0.5927, 16.8281) (-0.4192, 16.5995) (-0.2782, 16.5995) knots 0 0 0 1 2 2 2
  spline S181 degree 2 poles (-0.2782, 16.5995) (-0.1518, 16.5995) (-0.0011, 16.7341) (0.033, 16.8605) knots 0 0 0 1 2 2 2
  spline S182 degree 2 poles (0.033, 16.8605) (0.0556, 16.9447) (0.114, 17.1895) (0.1383, 17.2705) knots 0 0 0 1 2 2 2
  spline S183 degree 2 poles (0.1383, 17.2705) (0.2015, 17.4764) (0.456, 17.6676) (0.6424, 17.6676) knots 0 0 0 1 2 2 2
  spline S184 degree 2 poles (0.6424, 17.6676) (0.7607, 17.6676) (0.9876, 17.572) (1.067, 17.4861) knots 0 0 0 1 2 2 2
  spline S185 degree 2 poles (1.067, 17.4861) (1.1545, 17.3905) (1.2485, 17.1473) (1.2485, 16.9642) knots 0 0 0 1 2 2 2
  line L162 (1.2129, 19.0971) -> (1.2129, 17.9383)
  line L163 (1.2129, 17.9383) -> (-0.7871, 17.9383)
  line L164 (-0.7871, 17.9383) -> (-0.7871, 18.2041)
  line L165 (-0.7871, 18.2041) -> (0.9762, 18.2041)
  line L166 (0.9762, 18.2041) -> (0.9762, 19.0971)
  line L167 (0.9762, 19.0971) -> (1.2129, 19.0971)
  spline S186 degree 2 poles (1.2485, 20.0874) (1.2485, 19.8929) (1.1172, 19.5639) (0.9859, 19.4439) knots 0 0 0 1 2 2 2
  spline S187 degree 2 poles (0.9859, 19.4439) (0.8563, 19.324) (0.4673, 19.1927) (0.2145, 19.1927) knots 0 0 0 1 2 2 2
  spline S188 degree 2 poles (0.2145, 19.1927) (-0.0367, 19.1927) (-0.4095, 19.3208) (-0.5473, 19.4423) knots 0 0 0 1 2 2 2
  spline S189 degree 2 poles (-0.5473, 19.4423) (-0.6818, 19.5623) (-0.8228, 19.8896) (-0.8228, 20.0922) knots 0 0 0 1 2 2 2
  spline S190 degree 2 poles (-0.8228, 20.0922) (-0.8228, 20.1927) (-0.7936, 20.3694) (-0.7709, 20.4439) knots 0 0 0 1 2 2 2
  spline S191 degree 2 poles (-0.7709, 20.4439) (-0.7499, 20.5088) (-0.6899, 20.6433) (-0.6542, 20.7097) knots 0 0 0 1 2 2 2
  line L168 (-0.6542, 20.7097) -> (-0.3333, 20.7097)
  line L169 (-0.3333, 20.7097) -> (-0.3333, 20.6887)
  spline S192 degree 2 poles (-0.3333, 20.6887) (-0.3658, 20.653) (-0.4565, 20.5428) (-0.5003, 20.4634) knots 0 0 0 1 2 2 2
  spline S193 degree 2 poles (-0.5003, 20.4634) (-0.5424, 20.3872) (-0.5959, 20.2073) (-0.5959, 20.0906) knots 0 0 0 1 2 2 2
  spline S194 degree 2 poles (-0.5959, 20.0906) (-0.5959, 19.9626) (-0.4906, 19.7341) (-0.3901, 19.6482) knots 0 0 0 1 2 2 2
  spline S195 degree 2 poles (-0.3901, 19.6482) (-0.288, 19.5639) (0.0216, 19.4699) (0.2145, 19.4699) knots 0 0 0 1 2 2 2
  spline S196 degree 2 poles (0.2145, 19.4699) (0.4203, 19.4699) (0.7169, 19.5687) (0.819, 19.6546) knots 0 0 0 1 2 2 2
  spline S197 degree 2 poles (0.819, 19.6546) (0.9179, 19.7389) (1.0184, 19.9642) (1.0184, 20.0906) knots 0 0 0 1 2 2 2
  spline S198 degree 2 poles (1.0184, 20.0906) (1.0184, 20.2057) (0.9616, 20.4018) (0.9195, 20.478) knots 0 0 0 1 2 2 2
  spline S199 degree 2 poles (0.9195, 20.478) (0.8774, 20.5509) (0.7898, 20.6595) (0.759, 20.6903) knots 0 0 0 1 2 2 2
  line L170 (0.759, 20.6903) -> (0.759, 20.7097)
  line L171 (0.759, 20.7097) -> (1.0767, 20.7097)
  spline S200 degree 2 poles (1.0767, 20.7097) (1.1075, 20.6433) (1.1642, 20.5266) (1.1902, 20.4439) knots 0 0 0 1 2 2 2
  spline S201 degree 2 poles (1.1902, 20.4439) (1.2193, 20.3564) (1.2485, 20.2073) (1.2485, 20.0874) knots 0 0 0 1 2 2 2
  spline S202 degree 2 poles (-0.1842, 22.2219) (-0.0546, 22.2219) (0.1788, 22.1295) (0.2599, 22.0469) knots 0 0 0 1 2 2 2
  spline S203 degree 2 poles (0.2599, 22.0469) (0.362, 21.9431) (0.4673, 21.6627) (0.4673, 21.4488) knots 0 0 0 1 2 2 2
  line L172 (0.4673, 21.4488) -> (0.4673, 21.2235)
  line L173 (0.4673, 21.2235) -> (1.2129, 21.2235)
  line L174 (1.2129, 21.2235) -> (1.2129, 20.9577)
  line L175 (1.2129, 20.9577) -> (-0.7871, 20.9577)
  line L176 (-0.7871, 20.9577) -> (-0.7871, 21.4601)
  spline S204 degree 2 poles (-0.7871, 21.4601) (-0.7871, 21.6384) (-0.7288, 21.888) (-0.6623, 21.9836) knots 0 0 0 1 2 2 2
  spline S205 degree 2 poles (-0.6623, 21.9836) (-0.5862, 22.0955) (-0.3512, 22.2219) (-0.1842, 22.2219) knots 0 0 0 1 2 2 2
  spline S206 degree 2 poles (-0.1761, 21.9447) (-0.2799, 21.9447) (-0.4322, 21.8734) (-0.4808, 21.8005) knots 0 0 0 1 2 2 2
  spline S207 degree 2 poles (-0.4808, 21.8005) (-0.523, 21.7373) (-0.557, 21.5687) (-0.557, 21.4439) knots 0 0 0 1 2 2 2
  line L177 (-0.557, 21.4439) -> (-0.557, 21.2235)
  line L178 (-0.557, 21.2235) -> (0.2404, 21.2235)
  line L179 (0.2404, 21.2235) -> (0.2404, 21.405)
  spline S208 degree 2 poles (0.2404, 21.405) (0.2404, 21.5671) (0.1885, 21.7665) (0.1205, 21.8313) knots 0 0 0 1 2 2 2
  spline S209 degree 2 poles (0.1205, 21.8313) (0.0605, 21.8913) (-0.0805, 21.9447) (-0.1761, 21.9447) knots 0 0 0 1 2 2 2
  line L180 (1.2129, 24.8815) -> (1.2129, 24.5363)
  line L181 (1.2129, 24.5363) -> (0.4171, 23.9042)
  line L182 (0.4171, 23.9042) -> (0.4171, 23.5995)
  line L183 (0.4171, 23.5995) -> (1.2129, 23.5995)
  line L184 (1.2129, 23.5995) -> (1.2129, 23.3337)
  line L185 (1.2129, 23.3337) -> (-0.7871, 23.3337)
  line L186 (-0.7871, 23.3337) -> (-0.7871, 23.8491)
  spline S210 degree 2 poles (-0.7871, 23.8491) (-0.7871, 24.0209) (-0.7499, 24.2527) (-0.6818, 24.358) knots 0 0 0 1 2 2 2
  spline S211 degree 2 poles (-0.6818, 24.358) (-0.6137, 24.4634) (-0.4014, 24.5849) (-0.2442, 24.5849) knots 0 0 0 1 2 2 2
  spline S212 degree 2 poles (-0.2442, 24.5849) (-0.0254, 24.5849) (0.2712, 24.3613) (0.3425, 24.17) knots 0 0 0 1 2 2 2
  line L187 (0.3425, 24.17) -> (1.2129, 24.8815)
  spline S213 degree 2 poles (-0.2231, 24.3078) (-0.3106, 24.3078) (-0.4452, 24.2462) (-0.4889, 24.1814) knots 0 0 0 1 2 2 2
  spline S214 degree 2 poles (-0.4889, 24.1814) (-0.5262, 24.1247) (-0.557, 23.9739) (-0.557, 23.8637) knots 0 0 0 1 2 2 2
  line L188 (-0.557, 23.8637) -> (-0.557, 23.5995)
  line L189 (-0.557, 23.5995) -> (0.195, 23.5995)
  line L190 (0.195, 23.5995) -> (0.195, 23.8329)
  spline S215 degree 2 poles (0.195, 23.8329) (0.195, 23.948) (0.1545, 24.1311) (0.0913, 24.1943) knots 0 0 0 1 2 2 2
  spline S216 degree 2 poles (0.0913, 24.1943) (0.0362, 24.2527) (-0.1194, 24.3078) (-0.2231, 24.3078) knots 0 0 0 1 2 2 2
  line L191 (1.2129, 26.1165) -> (1.2129, 25.1409)
  line L192 (1.2129, 25.1409) -> (1.0086, 25.1409)
  line L193 (1.0086, 25.1409) -> (1.0086, 25.5039)
  line L194 (1.0086, 25.5039) -> (-0.3317, 25.5039)
  line L195 (-0.3317, 25.5039) -> (-0.3317, 25.1409)
  line L196 (-0.3317, 25.1409) -> (-0.5149, 25.1409)
  spline S217 degree 2 poles (-0.5149, 25.1409) (-0.5149, 25.3467) (-0.6316, 25.5412) (-0.7936, 25.5541) knots 0 0 0 1 2 2 2
  line L197 (-0.7936, 25.5541) -> (-0.7936, 25.7616)
  line L198 (-0.7936, 25.7616) -> (1.0086, 25.7616)
  line L199 (1.0086, 25.7616) -> (1.0086, 26.1165)
  line L200 (1.0086, 26.1165) -> (1.2129, 26.1165)
  spline S218 degree 2 poles (-0.1842, 28.6644) (-0.0546, 28.6644) (0.1788, 28.572) (0.2599, 28.4893) knots 0 0 0 1 2 2 2
  spline S219 degree 2 poles (0.2599, 28.4893) (0.362, 28.3856) (0.4673, 28.1052) (0.4673, 27.8913) knots 0 0 0 1 2 2 2
  line L201 (0.4673, 27.8913) -> (0.4673, 27.666)
  line L202 (0.4673, 27.666) -> (1.2129, 27.666)
  line L203 (1.2129, 27.666) -> (1.2129, 27.4002)
  line L204 (1.2129, 27.4002) -> (-0.7871, 27.4002)
  line L205 (-0.7871, 27.4002) -> (-0.7871, 27.9026)
  spline S220 degree 2 poles (-0.7871, 27.9026) (-0.7871, 28.0809) (-0.7288, 28.3305) (-0.6623, 28.4261) knots 0 0 0 1 2 2 2
  spline S221 degree 2 poles (-0.6623, 28.4261) (-0.5862, 28.5379) (-0.3512, 28.6644) (-0.1842, 28.6644) knots 0 0 0 1 2 2 2
  spline S222 degree 2 poles (-0.1761, 28.3872) (-0.2799, 28.3872) (-0.4322, 28.3159) (-0.4808, 28.243) knots 0 0 0 1 2 2 2
  spline S223 degree 2 poles (-0.4808, 28.243) (-0.523, 28.1798) (-0.557, 28.0112) (-0.557, 27.8864) knots 0 0 0 1 2 2 2
  line L206 (-0.557, 27.8864) -> (-0.557, 27.666)
  line L207 (-0.557, 27.666) -> (0.2404, 27.666)
  line L208 (0.2404, 27.666) -> (0.2404, 27.8475)
  spline S224 degree 2 poles (0.2404, 27.8475) (0.2404, 28.0096) (0.1885, 28.2089) (0.1205, 28.2738) knots 0 0 0 1 2 2 2
  spline S225 degree 2 poles (0.1205, 28.2738) (0.0605, 28.3337) (-0.0805, 28.3872) (-0.1761, 28.3872) knots 0 0 0 1 2 2 2
  spline S226 degree 2 poles (1.054, 29.7341) (1.0767, 29.7033) (1.1577, 29.5995) (1.1821, 29.5509) knots 0 0 0 1 2 2 2
  spline S227 degree 2 poles (1.1821, 29.5509) (1.2177, 29.4845) (1.255, 29.3597) (1.255, 29.2462) knots 0 0 0 1 2 2 2
  spline S228 degree 2 poles (1.255, 29.2462) (1.255, 29.1538) (1.1853, 28.9869) (1.1221, 28.9237) knots 0 0 0 1 2 2 2
  spline S229 degree 2 poles (1.1221, 28.9237) (1.0605, 28.8637) (0.879, 28.7908) (0.7785, 28.7908) knots 0 0 0 1 2 2 2
  spline S230 degree 2 poles (0.7785, 28.7908) (0.6229, 28.7908) (0.4025, 28.9221) (0.3393, 29.0647) knots 0 0 0 1 2 2 2
  spline S231 degree 2 poles (0.3393, 29.0647) (0.2809, 29.1911) (0.2372, 29.5347) (0.2258, 29.7341) knots 0 0 0 1 2 2 2
  line L209 (0.2258, 29.7341) -> (0.1772, 29.7341)
  spline S232 degree 2 poles (0.1772, 29.7341) (0.0897, 29.7341) (-0.0189, 29.6806) (-0.0497, 29.6319) knots 0 0 0 1 2 2 2
  spline S233 degree 2 poles (-0.0497, 29.6319) (-0.0805, 29.5833) (-0.1, 29.4439) (-0.1, 29.3694) knots 0 0 0 1 2 2 2
  spline S234 degree 2 poles (-0.1, 29.3694) (-0.1, 29.2819) (-0.0481, 29.0452) (0.0022, 28.9269) knots 0 0 0 1 2 2 2
  line L210 (0.0022, 28.9269) -> (0.0022, 28.9123)
  line L211 (0.0022, 28.9123) -> (-0.2555, 28.9123)
  spline S235 degree 2 poles (-0.2555, 28.9123) (-0.275, 28.982) (-0.3236, 29.243) (-0.3236, 29.371) knots 0 0 0 1 2 2 2
  spline S236 degree 2 poles (-0.3236, 29.371) (-0.3236, 29.5266) (-0.275, 29.7389) (-0.2118, 29.8232) knots 0 0 0 1 2 2 2
  spline S237 degree 2 poles (-0.2118, 29.8232) (-0.1502, 29.9058) (0.0459, 29.9869) (0.1869, 29.9869) knots 0 0 0 1 2 2 2
  line L212 (0.1869, 29.9869) -> (1.2129, 29.9869)
  line L213 (1.2129, 29.9869) -> (1.2129, 29.7341)
  line L214 (1.2129, 29.7341) -> (1.054, 29.7341)
  line L215 (0.8433, 29.7341) -> (0.4268, 29.7341)
  spline S238 degree 2 poles (0.4268, 29.7341) (0.4349, 29.6433) (0.4624, 29.3694) (0.4884, 29.2835) knots 0 0 0 1 2 2 2
  spline S239 degree 2 poles (0.4884, 29.2835) (0.5192, 29.183) (0.6472, 29.0517) (0.7607, 29.0517) knots 0 0 0 1 2 2 2
  spline S240 degree 2 poles (0.7607, 29.0517) (0.8903, 29.0517) (1.0216, 29.1976) (1.0216, 29.337) knots 0 0 0 1 2 2 2
  spline S241 degree 2 poles (1.0216, 29.337) (1.0216, 29.4553) (0.9195, 29.6498) (0.8433, 29.7341) knots 0 0 0 1 2 2 2
  line L216 (-0.0173, 31.1376) -> (-0.0173, 31.1247)
  spline S242 degree 2 poles (-0.0173, 31.1247) (-0.0254, 31.0955) (-0.0286, 31.0323) (-0.0286, 30.9885) knots 0 0 0 1 2 2 2
  spline S243 degree 2 poles (-0.0286, 30.9885) (-0.0286, 30.8864) (0.0605, 30.6854) (0.148, 30.5947) knots 0 0 0 1 2 2 2
  line L217 (0.148, 30.5947) -> (1.2129, 30.5947)
  line L218 (1.2129, 30.5947) -> (1.2129, 30.3418)
  line L219 (1.2129, 30.3418) -> (-0.288, 30.3418)
  line L220 (-0.288, 30.3418) -> (-0.288, 30.5947)
  line L221 (-0.288, 30.5947) -> (-0.0643, 30.5947)
  spline S244 degree 2 poles (-0.0643, 30.5947) (-0.1875, 30.7324) (-0.288, 30.9383) (-0.288, 31.0355) knots 0 0 0 1 2 2 2
  spline S245 degree 2 poles (-0.288, 31.0355) (-0.288, 31.0744) (-0.2847, 31.1133) (-0.2799, 31.1376) knots 0 0 0 1 2 2 2
  line L222 (-0.2799, 31.1376) -> (-0.0173, 31.1376)
  spline S246 degree 2 poles (1.242, 31.7875) (1.242, 31.5817) (1.007, 31.3499) (0.7526, 31.3499) knots 0 0 0 1 2 2 2
  line L223 (0.7526, 31.3499) -> (-0.0789, 31.3499)
  line L224 (-0.0789, 31.3499) -> (-0.0789, 31.1798)
  line L225 (-0.0789, 31.1798) -> (-0.288, 31.1798)
  line L226 (-0.288, 31.1798) -> (-0.288, 31.3499)
  line L227 (-0.288, 31.3499) -> (-0.7191, 31.3499)
  line L228 (-0.7191, 31.3499) -> (-0.7191, 31.6028)
  line L229 (-0.7191, 31.6028) -> (-0.288, 31.6028)
  line L230 (-0.288, 31.6028) -> (-0.288, 32.0679)
  line L231 (-0.288, 32.0679) -> (-0.0789, 32.0679)
  line L232 (-0.0789, 32.0679) -> (-0.0789, 31.6028)
  line L233 (-0.0789, 31.6028) -> (0.6359, 31.6028)
  spline S247 degree 2 poles (0.6359, 31.6028) (0.7493, 31.6028) (0.8741, 31.6109) (0.9276, 31.6384) knots 0 0 0 1 2 2 2
  spline S248 degree 2 poles (0.9276, 31.6384) (0.9746, 31.6611) (1.0216, 31.7632) (1.0216, 31.8507) knots 0 0 0 1 2 2 2
  spline S249 degree 2 poles (1.0216, 31.8507) (1.0216, 31.9123) (0.9843, 32.0274) (0.973, 32.0533) knots 0 0 0 1 2 2 2
  line L234 (0.973, 32.0533) -> (0.973, 32.0679)
  line L235 (0.973, 32.0679) -> (1.1999, 32.0679)
  spline S250 degree 2 poles (1.1999, 32.0679) (1.2193, 31.9966) (1.242, 31.8507) (1.242, 31.7875) knots 0 0 0 1 2 2 2
  spline S251 degree 2 poles (0.5986, 34.4893) (0.7477, 34.4893) (0.9762, 34.3759) (1.0508, 34.2819) knots 0 0 0 1 2 2 2
  spline S252 degree 2 poles (1.0508, 34.2819) (1.1383, 34.1684) (1.2129, 33.9107) (1.2129, 33.7065) knots 0 0 0 1 2 2 2
  line L236 (1.2129, 33.7065) -> (1.2129, 33.1328)
  line L237 (1.2129, 33.1328) -> (-0.7871, 33.1328)
  line L238 (-0.7871, 33.1328) -> (-0.7871, 33.6627)
  spline S253 degree 2 poles (-0.7871, 33.6627) (-0.7871, 33.8767) (-0.7596, 34.0906) (-0.7061, 34.1879) knots 0 0 0 1 2 2 2
  spline S254 degree 2 poles (-0.7061, 34.1879) (-0.6494, 34.2964) (-0.463, 34.3953) (-0.3366, 34.3953) knots 0 0 0 1 2 2 2
  spline S255 degree 2 poles (-0.3366, 34.3953) (-0.1956, 34.3953) (0.0281, 34.2462) (0.0913, 34.1149) knots 0 0 0 1 2 2 2
  line L239 (0.0913, 34.1149) -> (0.101, 34.1149)
  spline S256 degree 2 poles (0.101, 34.1149) (0.1496, 34.2932) (0.4073, 34.4893) (0.5986, 34.4893) knots 0 0 0 1 2 2 2
  spline S257 degree 2 poles (0.6099, 34.2122) (0.4965, 34.2122) (0.3506, 34.1473) (0.2988, 34.0501) knots 0 0 0 1 2 2 2
  spline S258 degree 2 poles (0.2988, 34.0501) (0.2663, 33.9869) (0.2469, 33.8378) (0.2469, 33.7) knots 0 0 0 1 2 2 2
  line L240 (0.2469, 33.7) -> (0.2469, 33.3986)
  line L241 (0.2469, 33.3986) -> (0.9859, 33.3986)
  line L242 (0.9859, 33.3986) -> (0.9859, 33.6141)
  spline S259 degree 2 poles (0.9859, 33.6141) (0.9859, 33.7892) (0.9535, 33.9901) (0.9017, 34.0679) knots 0 0 0 1 2 2 2
  spline S260 degree 2 poles (0.9017, 34.0679) (0.8482, 34.1425) (0.7153, 34.2122) (0.6099, 34.2122) knots 0 0 0 1 2 2 2
  spline S261 degree 2 poles (-0.2993, 34.1182) (-0.3706, 34.1182) (-0.4776, 34.0695) (-0.5084, 34.0161) knots 0 0 0 1 2 2 2
  spline S262 degree 2 poles (-0.5084, 34.0161) (-0.544, 33.9512) (-0.5602, 33.794) (-0.5602, 33.653) knots 0 0 0 1 2 2 2
  line L243 (-0.5602, 33.653) -> (-0.5602, 33.3986)
  line L244 (-0.5602, 33.3986) -> (0.0248, 33.3986)
  line L245 (0.0248, 33.3986) -> (0.0248, 33.7)
  spline S263 degree 2 poles (0.0248, 33.7) (0.0248, 33.8248) (-0.0011, 33.9431) (-0.0416, 34.0063) knots 0 0 0 1 2 2 2
  spline S264 degree 2 poles (-0.0416, 34.0063) (-0.0805, 34.0679) (-0.2053, 34.1182) (-0.2993, 34.1182) knots 0 0 0 1 2 2 2
  spline S265 degree 2 poles (1.054, 35.5704) (1.0767, 35.5396) (1.1577, 35.4358) (1.1821, 35.3872) knots 0 0 0 1 2 2 2
  spline S266 degree 2 poles (1.1821, 35.3872) (1.2177, 35.3208) (1.255, 35.196) (1.255, 35.0825) knots 0 0 0 1 2 2 2
  spline S267 degree 2 poles (1.255, 35.0825) (1.255, 34.9901) (1.1853, 34.8232) (1.1221, 34.76) knots 0 0 0 1 2 2 2
  spline S268 degree 2 poles (1.1221, 34.76) (1.0605, 34.7) (0.879, 34.6271) (0.7785, 34.6271) knots 0 0 0 1 2 2 2
  spline S269 degree 2 poles (0.7785, 34.6271) (0.6229, 34.6271) (0.4025, 34.7584) (0.3393, 34.901) knots 0 0 0 1 2 2 2
  spline S270 degree 2 poles (0.3393, 34.901) (0.2809, 35.0274) (0.2372, 35.371) (0.2258, 35.5704) knots 0 0 0 1 2 2 2
  line L246 (0.2258, 35.5704) -> (0.1772, 35.5704)
  spline S271 degree 2 poles (0.1772, 35.5704) (0.0897, 35.5704) (-0.0189, 35.5169) (-0.0497, 35.4682) knots 0 0 0 1 2 2 2
  spline S272 degree 2 poles (-0.0497, 35.4682) (-0.0805, 35.4196) (-0.1, 35.2802) (-0.1, 35.2057) knots 0 0 0 1 2 2 2
  spline S273 degree 2 poles (-0.1, 35.2057) (-0.1, 35.1182) (-0.0481, 34.8815) (0.0022, 34.7632) knots 0 0 0 1 2 2 2
  line L247 (0.0022, 34.7632) -> (0.0022, 34.7486)
  line L248 (0.0022, 34.7486) -> (-0.2555, 34.7486)
  spline S274 degree 2 poles (-0.2555, 34.7486) (-0.275, 34.8183) (-0.3236, 35.0793) (-0.3236, 35.2073) knots 0 0 0 1 2 2 2
  spline S275 degree 2 poles (-0.3236, 35.2073) (-0.3236, 35.3629) (-0.275, 35.5752) (-0.2118, 35.6595) knots 0 0 0 1 2 2 2
  spline S276 degree 2 poles (-0.2118, 35.6595) (-0.1502, 35.7422) (0.0459, 35.8232) (0.1869, 35.8232) knots 0 0 0 1 2 2 2
  line L249 (0.1869, 35.8232) -> (1.2129, 35.8232)
  line L250 (1.2129, 35.8232) -> (1.2129, 35.5704)
  line L251 (1.2129, 35.5704) -> (1.054, 35.5704)
  line L252 (0.8433, 35.5704) -> (0.4268, 35.5704)
  spline S277 degree 2 poles (0.4268, 35.5704) (0.4349, 35.4796) (0.4624, 35.2057) (0.4884, 35.1198) knots 0 0 0 1 2 2 2
  spline S278 degree 2 poles (0.4884, 35.1198) (0.5192, 35.0193) (0.6472, 34.888) (0.7607, 34.888) knots 0 0 0 1 2 2 2
  spline S279 degree 2 poles (0.7607, 34.888) (0.8903, 34.888) (1.0216, 35.0339) (1.0216, 35.1733) knots 0 0 0 1 2 2 2
  spline S280 degree 2 poles (1.0216, 35.1733) (1.0216, 35.2916) (0.9195, 35.4861) (0.8433, 35.5704) knots 0 0 0 1 2 2 2
  spline S281 degree 2 poles (1.2485, 36.5833) (1.2485, 36.4326) (1.1675, 36.1717) (1.1221, 36.0858) knots 0 0 0 1 2 2 2
  line L253 (1.1221, 36.0858) -> (0.8385, 36.0858)
  line L254 (0.8385, 36.0858) -> (0.8385, 36.0987)
  spline S282 degree 2 poles (0.8385, 36.0987) (0.8644, 36.1311) (0.926, 36.2187) (0.96, 36.2916) knots 0 0 0 1 2 2 2
  spline S283 degree 2 poles (0.96, 36.2916) (0.9908, 36.3548) (1.0362, 36.5104) (1.0362, 36.593) knots 0 0 0 1 2 2 2
  spline S284 degree 2 poles (1.0362, 36.593) (1.0362, 36.653) (1.0086, 36.7908) (0.9859, 36.8232) knots 0 0 0 1 2 2 2
  spline S285 degree 2 poles (0.9859, 36.8232) (0.9552, 36.8702) (0.8855, 36.9123) (0.8141, 36.9123) knots 0 0 0 1 2 2 2
  spline S286 degree 2 poles (0.8141, 36.9123) (0.725, 36.9123) (0.6326, 36.8151) (0.6018, 36.6903) knots 0 0 0 1 2 2 2
  spline S287 degree 2 poles (0.6018, 36.6903) (0.5905, 36.6417) (0.5581, 36.4861) (0.5402, 36.4196) knots 0 0 0 1 2 2 2
  spline S288 degree 2 poles (0.5402, 36.4196) (0.49, 36.2478) (0.2825, 36.0922) (0.1351, 36.0922) knots 0 0 0 1 2 2 2
  spline S289 degree 2 poles (0.1351, 36.0922) (-0.0692, 36.0922) (-0.3236, 36.3986) (-0.3236, 36.6514) knots 0 0 0 1 2 2 2
  spline S290 degree 2 poles (-0.3236, 36.6514) (-0.3236, 36.7762) (-0.262, 37.029) (-0.215, 37.1149) knots 0 0 0 1 2 2 2
  line L255 (-0.215, 37.1149) -> (0.0556, 37.1149)
  line L256 (0.0556, 37.1149) -> (0.0556, 37.102)
  spline S291 degree 2 poles (0.0556, 37.102) (-0.0222, 37.0047) (-0.1113, 36.7681) (-0.1113, 36.6465) knots 0 0 0 1 2 2 2
  spline S292 degree 2 poles (-0.1113, 36.6465) (-0.1113, 36.5217) (-0.0059, 36.3499) (0.0994, 36.3499) knots 0 0 0 1 2 2 2
  spline S293 degree 2 poles (0.0994, 36.3499) (0.195, 36.3499) (0.2874, 36.452) (0.3166, 36.5655) knots 0 0 0 1 2 2 2
  spline S294 degree 2 poles (0.3166, 36.5655) (0.3312, 36.6206) (0.3603, 36.76) (0.3782, 36.8362) knots 0 0 0 1 2 2 2
  spline S295 degree 2 poles (0.3782, 36.8362) (0.4203, 37.0015) (0.6132, 37.17) (0.7801, 37.17) knots 0 0 0 1 2 2 2
  spline S296 degree 2 poles (0.7801, 37.17) (0.8774, 37.17) (1.0492, 37.0939) (1.1124, 37.0193) knots 0 0 0 1 2 2 2
  spline S297 degree 2 poles (1.1124, 37.0193) (1.1788, 36.9399) (1.2485, 36.7373) (1.2485, 36.5833) knots 0 0 0 1 2 2 2
  spline S298 degree 2 poles (1.2469, 38.0566) (1.2469, 37.6968) (0.8433, 37.3013) (0.4706, 37.3013) knots 0 0 0 1 2 2 2